Autodesk Fusion 360 part; units mm, degrees
(part 2 of 2)
sketch "Sketch1" plane through (0, 0, 0) normal (0, 0, 1) x (1, 0, 0) in component "Up  Cover - Back"
  line L0 (64, 138) -> (-64, 138)
  line L1 (-64, 138) -> (-64, -138)
  line L2 (-64, -138) -> (64, -138)
  line L3 (64, -138) -> (64, 138)
  line L4 (64, 138) -> (-64, -138) construction
  line L5 (-64, 138) -> (64, -138) construction
  line L6 (-64, 138) -> (-74, 138)
  line L7 (-74, 138) -> (-74, -138)
  line L8 (-74, -138) -> (-64, -138)
  line L9 (-64, -138) -> (-64, 138)
  line L10 (64, 138) -> (87.5, 138)
  line L11 (87.5, 138) -> (87.5, -138)
  line L12 (87.5, -138) -> (64, -138)
  line L13 (64, -138) -> (64, 138)
  circle A0 centre (-74, 0) radius 15
  line L14 (14, 138) -> (64, 88)
  line L15 (64, -88) -> (14, -138)
  line L16 (-74, -138) -> (87.5, -138)
  line L17 (87.5, -138) -> (87.5, -162)
  line L18 (87.5, -162) -> (-74, -162)
  line L19 (-74, -162) -> (-74, -138)
  line L20 (-74, 138) -> (87.5, 138)
  line L21 (87.5, 138) -> (87.5, 162)
  line L22 (87.5, 162) -> (-74, 162)
  line L23 (-74, 162) -> (-74, 138)
  dimension "d3" = 10
  dimension "d4" = 23.5
  dimension "d5" = 30
  dimension "d6" = 50
  dimension "d7" = 50
  dimension "d8" = 50
  dimension "d9" = 50
  dimension "d14" = 161.5
  dimension "d15" = 24
  dimension "d16" = 24
  dimension "d17" = 324
  constraint horizontal L0
  constraint perpendicular L0 L1
  constraint parallel L0 L2
  constraint parallel L1 L3
  constraint coincident L4 origin
  constraint coincident L5 origin
  constraint horizontal L6
  constraint vertical L7
  constraint horizontal L8
  constraint vertical L9
  constraint coincident L1.end L2.start
  constraint horizontal L10
  constraint vertical L11
  constraint horizontal L12
  constraint vertical L13
  constraint coincident L2.end L3.start
  constraint midpoint L7 A0.centre
  constraint coincident L0 L14.start
  constraint coincident L3 L14.end
  constraint coincident L3 L15.start
  constraint coincident L2 L15.end
  constraint horizontal L16
  constraint vertical L17
  constraint horizontal L18
  constraint vertical L19
  constraint coincident L11.end L12.start
  constraint horizontal L20
  constraint vertical L21
  constraint horizontal L22
  constraint vertical L23
  constraint coincident L10.end L11.start
  measures "d3" distance of L0.end L6.end
  measures "d4" distance of L0.start L10.end
  measures "d5" diameter of A0
  measures "d6" distance of L2.end L15.end
  measures "d7" distance of L2.end L15.start
  measures "d8" distance of L0.start L14.end
  measures "d9" distance of L0.start L14.start
  measures "d14" distance of L6.end L10.end
  measures "d15" distance of L11.end L17.end
  measures "d16" distance of L10.end L21.end
  measures "d17" distance of L18.end L22.end
extrude "Extrude1" add sketch "Sketch1" against normal blind 3 contours L0 L3 L13 L14 L20 | L3 L10 L11 L12 L13 L16 L20 | L0 L6 L10 L20 L21 L22 L23 | L0 L1 L2 L3 L9 L13 A0 L14 L15 L16 L20 | L1 L6 L7 L9 A0 L20 | L2 L3 L13 L15 L16 | L2 L8 L12 L16 L17 L18 L19 | L1 L7 L8 L9 A0 L16 makes body 1 in component "Up  Cover - Back"
extrude "Extrude2" add sketch "Sketch1" along normal blind 5 contours L0 L1 L2 L3 L9 L13 A0 L14 L15 L16 L20 bodies 1 in component "Up  Cover - Back"
sketch "Sketch2" plane through (0, 0, 5) normal (0, 0, 1) x (-1, 0, 0) in component "Up  Cover - Back"
  line L0 (-14, -138) -> (64, -138)
  line L1 (64, -138) -> (64, -11.1803)
  arc A0 (64, 11.1803) -> (64, -11.1803) centre (74, 0) ccw
  line L2 (64, 11.1803) -> (64, 138)
  line L3 (64, 138) -> (-14, 138)
  line L4 (-14, 138) -> (-64, 88)
  line L5 (-64, 88) -> (-64, -88)
  line L6 (-64, -88) -> (-14, -138)
  line L7 (59.8579, -5) -> (-64, -5)
  line L8 (59.8579, 5) -> (-64, 5)
  line L9 (-64, -5) -> (-60, -5)
  line L10 (-60, -5) -> (-60, -25)
  line L11 (-60, -25) -> (-64, -25)
  line L12 (-64, -25) -> (-64, -5)
  line L13 (59.8579, -5) -> (55.8579, -5)
  line L14 (55.8579, -5) -> (55.8579, -25)
  line L15 (55.8579, -25) -> (59.8579, -25)
  line L16 (59.8579, -25) -> (59.8579, -5)
  line L17 (55.8579, -15) -> (-60, -15) construction
  line L18 (-4.0711, -5) -> (-0.0711, -5)
  line L19 (-0.0711, -5) -> (-0.0711, -25)
  line L20 (-0.0711, -25) -> (-4.0711, -25)
  line L21 (-4.0711, -25) -> (-4.0711, -5)
  line L22 (-4.0711, -5) -> (-0.0711, -25) construction
  line L23 (-0.0711, -5) -> (-4.0711, -25) construction
  line L24 (59, 0) -> (-64, 0) construction
  line L25 (59.8579, 5) -> (55.8579, 5)
  line L26 (55.8579, 25) -> (59.8579, 25)
  line L27 (59.8579, 25) -> (59.8579, 5)
  line L28 (55.8579, 5) -> (55.8579, 25)
  line L29 (-0.0711, 5) -> (-0.0711, 25)
  line L30 (-0.0711, 25) -> (-4.0711, 25)
  line L31 (-4.0711, 5) -> (-0.0711, 5)
  line L32 (-4.0711, 25) -> (-4.0711, 5)
  line L33 (-64, 5) -> (-60, 5)
  line L34 (-60, 25) -> (-64, 25)
  line L35 (-64, 25) -> (-64, 5)
  line L36 (-60, 5) -> (-60, 25)
  point P0 (-2.0711, -15)
  dimension "d18" = 5
  dimension "d19" = 5
  dimension "d20" = 20
  dimension "d21" = 4
  dimension "d22" = 4
  dimension "d23" = 20
  dimension "d24" = 4
  dimension "d25" = 20
  constraint coincident A0 L7.start
  constraint coincident L5 L7.end
  constraint perpendicular L5 L7
  constraint coincident A0 L8.start
  constraint coincident L5 L8.end
  constraint perpendicular L5 L8
  constraint horizontal L9
  constraint vertical L10
  constraint horizontal L11
  constraint vertical L12
  constraint horizontal L13
  constraint vertical L14
  constraint horizontal L15
  constraint vertical L16
  constraint midpoint L14 L17.start
  constraint midpoint L10 L17.end
  constraint horizontal L18
  constraint perpendicular L18 L19
  constraint parallel L18 L20
  constraint parallel L19 L21
  constraint coincident L22 P0
  constraint coincident L23 P0
  constraint midpoint L17 P0
  constraint midpoint A0 L24.start
  constraint midpoint L5 L24.end
  constraint symmetric L7.start L24 L8.start
  constraint symmetric L7.end L24 L8.end
  constraint symmetric L9.end L24 L33.end
  constraint symmetric L10.end L24 L34.start
  constraint symmetric L11.end L24 L34.end
  constraint symmetric L13.end L24 L25.end
  constraint symmetric L14.end L24 L26.start
  constraint symmetric L15.end L24 L26.end
  constraint symmetric L18.start L24 L31.start
  constraint symmetric L18.end L24 L29.start
  constraint symmetric L19.end L24 L29.end
  constraint symmetric L20.end L24 L30.end
  measures "d18" vertical distance of origin L8.end
  measures "d19" vertical distance of origin L7.end
  measures "d20" distance of L7.end L11.end
  measures "d21" distance of L10.end L11.end
  measures "d22" distance of L7.start L13.end
  measures "d23" distance of L7.start L15.end
  measures "d24" distance of L19.end L20.end
  measures "d25" distance of L18.end L19.end
extrude "Extrude3" add sketch "Sketch2" along normal blind 20 contours L5 L7 L9 L10 L11 L12 | A0 L5 L7 L8 L9 L13 L18 L25 L31 L33 | L7 L13 L14 L15 L16 | L8 L25 L26 L27 L28 | L5 L8 L33 L34 L35 L36 | L7 L18 L19 L20 L21 | L8 L29 L30 L31 L32 bodies 1 in component "Up  Cover - Back"
chamfer "Chamfer1" distance 20 angle 45 6 edges at (-57.8579, -25, 25) (-57.8579, 25, 25) (2.0711, -25, 25) (2.0711, 25, 25) (62, 25, 25) (62, -25, 25) on bodies 1 in component "Up  Cover - Back"
sketch "Sketch3" plane through (0, -5, 0) normal (0, -1, 0) x (1, 0, 0) in component "Up  Cover - Back"
  line L0 (-55.8579, 5) -> (0.0711, 5)
  line L1 (0.0711, 5) -> (0.0711, 25)
  line L2 (0.0711, 25) -> (-55.8579, 25)
  line L3 (-55.8579, 25) -> (-55.8579, 5)
  line L4 (4.0711, 5) -> (60, 5)
  line L5 (60, 5) -> (60, 25)
  line L6 (60, 25) -> (4.0711, 25)
  line L7 (4.0711, 25) -> (4.0711, 5)
  line L8 (-55.8579, 15) -> (60, 15) construction
  circle A0 centre (-49.8579, 15) radius 2.1
  circle A1 centre (-15.8579, 15) radius 2.1
  circle A2 centre (20, 15) radius 2.1
  line L9 (32.0355, 25) -> (32.0355, 5) construction
  line L10 (-27.8934, 25) -> (-27.8934, 5) construction
  circle A3 centre (54, 15) radius 2.1
  line L11 (-59.8579, 25) -> (-59.8579, 5)
  line L12 (64, 5) -> (64, 25)
  dimension "d29" = 4.2
  dimension "d30" = 4.2
  dimension "d31" = 4.2
  dimension "d32" = 4.2
  dimension "d33" = 10
  dimension "d34" = 10
  dimension "d35" = 34
  dimension "d36" = 34
  constraint midpoint L3 L8.start
  constraint midpoint L5 L8.end
  constraint coincident L8 A0.centre
  constraint coincident L8 A1.centre
  constraint coincident L8 A2.centre
  constraint midpoint L6 L9.start
  constraint midpoint L4 L9.end
  constraint midpoint L2 L10.start
  constraint midpoint L0 L10.end
  constraint coincident L8 A3.centre
  measures "d29" diameter of A0
  measures "d30" diameter of A1
  measures "d32" diameter of A3
  measures "d33" distance of A0.centre L11
  measures "d34" distance of A3.centre L12
  measures "d35" distance of A0.centre A1.centre
  measures "d36" distance of A2.centre A3.centre
extrude "Extrude4" cut sketch "Sketch3" against normal through all contours A0 | A1 | A2 | A3 bodies 1 in component "Up  Cover - Back"
split "Split1" by plane through (0, 0, 0) normal (0, 1, 0) bodies 1 makes body 2 at (-16.8924, 111.7787, -3) in component "Up  Cover - Back"
component "Up  Cover - Back" placed x (1, 0, 0) y (0, 1, 0) z (0, 0, 1) at (0, 0, 0)
named bodies: "Up  Cover - Back Right", "Up  Cover - Back Left"

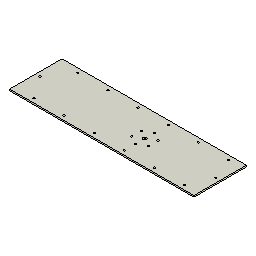
design "Side Cover"
Autodesk Fusion 360 part; units mm, degrees
sketch "Sketch2" plane through (0, 0, 0) normal (0, 0, 1) x (1, 0, 0)
  line L0 (-214.5, -61) -> (-214.5, 61)
  line L1 (-214.5, -61) -> (214.5, 61) construction
  line L2 (-214.5, 61) -> (214.5, 61)
  circle A0 centre (42.5, -3.3) radius 4.1
  line L3 (214.5, -61) -> (-214.5, 61) construction
  line L4 (214.5, 61) -> (214.5, -61)
  line L5 (214.5, -61) -> (-214.5, -61)
  line L6 (-214.5, 0) -> (214.5, 0) construction
  line L7 (-214.5, -3.3) -> (214.5, -3.3) construction
  line L8 (42.5, 61) -> (42.5, -61) construction
  circle A1 centre (42.5, 51) radius 2.1
  line L9 (-214.5, 51) -> (214.5, 51) construction
  circle A2 centre (42.5, -3.3) radius 22.5 construction
  circle A3 centre (42.5, 19.2) radius 2.1
  circle A4 centre (23.0144, 7.95) radius 2.1
  circle A5 centre (23.0144, -14.55) radius 2.1
  circle A6 centre (42.5, -25.8) radius 2.1
  circle A7 centre (61.9856, -14.55) radius 2.1
  circle A8 centre (61.9856, 7.95) radius 2.1
  line L10 (-194.5, 61) -> (-194.5, -61) construction
  line L11 (194.5, 61) -> (194.5, -61) construction
  circle A9 centre (-167.5, 51) radius 2.1
  circle A10 centre (-97.5, 51) radius 2.1
  circle A11 centre (-27.5, 51) radius 2.1
  circle A12 centre (112.5, 51) radius 2.1
  circle A13 centre (182.5, 51) radius 2.1
  circle A14 centre (112.5, -51) radius 2.1
  line L12 (-214.5, -51) -> (214.5, -51) construction
  circle A15 centre (-27.5, -51) radius 2.1
  circle A16 centre (-167.5, -51) radius 2.1
  circle A17 centre (182.5, -51) radius 2.1
  circle A18 centre (-97.5, -51) radius 2.1
  circle A19 centre (42.5, -51) radius 2.1
  circle A20 centre (-204.5, 0) radius 2.1
  circle A21 centre (204.5, 0) radius 2.1
  dimension "d11" = 122
  dimension "d12" = 429
  dimension "d14" = 8.2
  dimension "d18" = 3.3
  dimension "d20" = 172
  dimension "d21" = 4.2
  dimension "d23" = 10
  dimension "d24" = 45
  dimension "d25" = 4.2
  dimension "d27" = 360
  dimension "d30" = 70
  dimension "d31" = 0
  dimension "d32" = 20
  dimension "d33" = 20
  dimension "d34" = 4.2
  dimension "d35" = 10
  dimension "d36" = 4.2
  dimension "d37" = 10
  constraint perpendicular L0 L5
  constraint parallel L2 L5
  constraint parallel L0 L4
  constraint horizontal L5
  constraint coincident origin L3
  constraint coincident origin L1
  constraint midpoint L0 L6.start
  constraint midpoint L4 L6.end
  constraint coincident A0.centre L7
  constraint coincident L2 L8.start
  constraint coincident L5 L8.end
  constraint perpendicular L5 L8
  constraint coincident A0.centre L8
  constraint coincident L8 A1.centre
  constraint coincident L0 L9.start
  constraint coincident L4 L9.end
  constraint perpendicular L4 L9
  constraint coincident A1.centre L9
  constraint concentric A0 A2
  constraint coincident A2 A3.centre
  constraint coincident L8 A3.centre
  constraint coincident L2 L10.start
  constraint coincident L5 L10.end
  constraint perpendicular L5 L10
  constraint coincident L2 L11.start
  constraint coincident L5 L11.end
  constraint perpendicular L5 L11
  constraint symmetric L6 A1 A19
  constraint symmetric L6 L9.start L12.start
  constraint symmetric L6 L9.end L12.end
  constraint symmetric L6 A9 A16
  constraint symmetric L6 A10 A18
  constraint symmetric L6 A11 A15
  constraint symmetric L6 A12 A14
  constraint symmetric L6 A13 A17
  constraint coincident L6 A20.centre
  constraint coincident L6 A21.centre
  measures "d11" distance of L0.start L0.end
  measures "d12" distance of L0.end L1.end
  measures "d14" diameter of A0
  measures "d20" distance of L1.end L8.start
  measures "d21" diameter of A1
  measures "d23" distance of L1.end L9.end
  measures "d24" diameter of A2
  measures "d25" diameter of A3
  measures "d32" distance of L0 L10
  measures "d33" distance of L4 L11
  measures "d34" diameter of A20
  measures "d35" distance of L6.start A20.centre
  measures "d36" diameter of A21
  measures "d37" distance of L6.end A21.centre
extrude "Extrude2" add sketch "Sketch2" along normal blind 3.5
sketch "Sketch3" plane through (0, 0, 3.5) normal (0, 0, 1) x (-1, 0, 0)
  circle A0 centre (-42.5, 3.3) radius 4
  line L0 (-214.5, 61) -> (-214.5, -61)
  line L1 (-214.5, -61) -> (214.5, -61)
  line L2 (214.5, -61) -> (214.5, 61)
  line L3 (214.5, 61) -> (-214.5, 61)
  line L4 (-130, -50) -> (-141.5967, -50) construction
  line L5 (-141.5967, -50) -> (-141.5967, -60) construction
  line L6 (-141.5967, -60) -> (-130, -60) construction
  line L7 (-130, -60) -> (-130, -50) construction
  circle A1 centre (-182.5, 51) radius 2.1
  circle A2 centre (97.5, 51) radius 2.1
  circle A3 centre (-42.5, 51) radius 2.1
  circle A4 centre (204.5, 0) radius 2.1
  circle A5 centre (-204.5, 0) radius 2.1
  circle A6 centre (167.5, 51) radius 2.1
  circle A7 centre (97.5, -51) radius 2.1
  circle A8 centre (27.5, -51) radius 2.1
  circle A9 centre (-112.5, -51) radius 2.1
  circle A10 centre (-182.5, -51) radius 2.1
  circle A11 centre (-112.5, 51) radius 2.1
  circle A12 centre (27.5, 51) radius 2.1
  circle A13 centre (167.5, -51) radius 2.1
  circle A14 centre (-61.9856, -7.95) radius 2.1
  circle A15 centre (-61.9856, 14.55) radius 2.1
  circle A16 centre (-42.5, 25.8) radius 2.1
  circle A17 centre (-23.0144, 14.55) radius 2.1
  circle A18 centre (-23.0144, -7.95) radius 2.1
  circle A19 centre (-42.5, -19.2) radius 2.1
  circle A20 centre (-42.5, -51) radius 2.1
  circle A21 centre (-42.5, 3.3) radius 4.1
  line L8 (-214.5, 61) -> (-214.5, -61)
  line L9 (-214.5, -61) -> (214.5, -61)
  line L10 (214.5, -61) -> (214.5, 61)
  line L11 (214.5, 61) -> (-214.5, 61)
  constraint perpendicular L4 L5
  constraint parallel L4 L6
  constraint parallel L5 L7

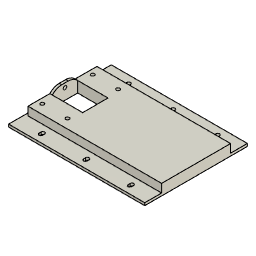
design "Back Cover"
Autodesk Fusion 360 part; units mm, degrees
sketch "Sketch1" plane through (0, 0, 0) normal (0, 0, 1) x (1, 0, 0)
  line L0 (-79.25, 60.9) -> (79.25, 60.9)
  line L1 (79.25, 60.9) -> (79.25, -60.9)
  line L2 (79.25, -60.9) -> (-79.25, -60.9)
  line L3 (-79.25, -60.9) -> (-79.25, 60.9)
  line L4 (-79.25, 60.9) -> (79.25, -60.9) construction
  line L5 (79.25, 60.9) -> (-79.25, -60.9) construction
  line L6 (79.25, -40.9) -> (-79.25, -40.9)
  line L7 (-79.25, -40.9) -> (-79.25, 40.9)
  line L8 (-79.25, 40.9) -> (79.25, 40.9)
  line L9 (79.25, 40.9) -> (79.25, -40.9)
  line L10 (79.25, -40.9) -> (-79.25, 40.9) construction
  line L11 (-79.25, -40.9) -> (79.25, 40.9) construction
  line L12 (0, 0) -> (0, 60.9) construction
  line L13 (-79.25, 60.9) -> (79.25, 40.9) construction
  line L14 (0, 50.9) -> (-79.25, 50.9) construction
  line L15 (0, 50.9) -> (79.25, 50.9) construction
  line L16 (-2.1, 52.15) -> (-2.1, 49.65)
  arc A0 (-2.1, 49.65) -> (2.1, 49.65) centre (0, 49.65) ccw
  line L17 (2.1, 49.65) -> (2.1, 52.15)
  arc A1 (2.1, 52.15) -> (-2.1, 52.15) centre (0, 52.15) ccw
  line L18 (0, 52.15) -> (0, 49.65) construction
  arc A2 (-50.7333, 52.15) -> (-54.9333, 52.15) centre (-52.8333, 52.15) ccw
  line L19 (-54.9333, 52.15) -> (-54.9333, 49.65)
  arc A3 (-54.9333, 49.65) -> (-50.7333, 49.65) centre (-52.8333, 49.65) ccw
  line L20 (-50.7333, 49.65) -> (-50.7333, 52.15)
  arc A4 (54.9333, 52.15) -> (50.7333, 52.15) centre (52.8333, 52.15) ccw
  line L21 (50.7333, 52.15) -> (50.7333, 49.65)
  arc A5 (50.7333, 49.65) -> (54.9333, 49.65) centre (52.8333, 49.65) ccw
  line L22 (54.9333, 49.65) -> (54.9333, 52.15)
  line L23 (-79.25, 0) -> (79.25, 0) construction
  arc A6 (-54.9333, -52.15) -> (-50.7333, -52.15) centre (-52.8333, -52.15) ccw
  line L24 (-54.9333, -52.15) -> (-54.9333, -49.65)
  arc A7 (-50.7333, -49.65) -> (-54.9333, -49.65) centre (-52.8333, -49.65) ccw
  line L25 (-50.7333, -49.65) -> (-50.7333, -52.15)
  arc A8 (-2.1, -52.15) -> (2.1, -52.15) centre (0, -52.15) ccw
  line L26 (-2.1, -52.15) -> (-2.1, -49.65)
  line L27 (2.1, -49.65) -> (2.1, -52.15)
  arc A9 (2.1, -49.65) -> (-2.1, -49.65) centre (0, -49.65) ccw
  arc A10 (50.7333, -52.15) -> (54.9333, -52.15) centre (52.8333, -52.15) ccw
  line L28 (50.7333, -52.15) -> (50.7333, -49.65)
  line L29 (54.9333, -49.65) -> (54.9333, -52.15)
  arc A11 (54.9333, -49.65) -> (50.7333, -49.65) centre (52.8333, -49.65) ccw
  line L30 (-2.1, 50.9) -> (2.1, 50.9) construction
  line L31 (-37.25, 40.9) -> (-37.25, -40.9) construction
  line L32 (-40.25, 15) -> (-76.25, 15)
  line L33 (-76.25, 15) -> (-76.25, -15)
  line L34 (-76.25, -15) -> (-40.25, -15)
  line L35 (-40.25, -15) -> (-40.25, 15)
  line L36 (-40.25, 15) -> (-76.25, -15) construction
  line L37 (-76.25, 15) -> (-40.25, -15) construction
  line L38 (-43.25, -30) -> (-73.25, -30) construction
  line L39 (-73.25, -30) -> (-73.25, 30) construction
  line L40 (-73.25, 30) -> (-43.25, 30) construction
  line L41 (-43.25, 30) -> (-43.25, -30) construction
  line L42 (-43.25, -30) -> (-73.25, 30) construction
  line L43 (-73.25, -30) -> (-43.25, 30) construction
  circle A12 centre (-73.25, -30) radius 2.1
  circle A13 centre (-43.25, -30) radius 2.1
  circle A14 centre (-73.25, 30) radius 2.1
  circle A15 centre (-43.25, 30) radius 2.1
  line L44 (-79.25, 60.9) -> (-82.25, 60.9)
  line L45 (-82.25, 60.9) -> (-82.25, -60.9)
  line L46 (-82.25, -60.9) -> (-79.25, -60.9)
  line L47 (-79.25, -60.9) -> (-79.25, 60.9)
  point P0 (-58.25, 0)
  point P1 (-58.25, 0)
  dimension "d1" = 121.8
  dimension "d2" = 158.5
  dimension "d3" = 81.8
  dimension "d13" = 4.2
  dimension "d14" = 2.5
  dimension "d22" = 52.8333
  dimension "d23" = 0
  dimension "d26" = 42
  dimension "d27" = 36
  dimension "d28" = 30
  dimension "d29" = 3
  dimension "d30" = 30
  dimension "d31" = 60
  dimension "d32" = 4.2
  dimension "d33" = 4.2
  dimension "d34" = 4.2
  dimension "d35" = 4.2
  dimension "d40" = 3
  constraint perpendicular L0 L1
  constraint parallel L0 L2
  constraint perpendicular L6 L7
  constraint parallel L6 L8
  constraint horizontal L6
  constraint coincident L1 L6.start
  constraint midpoint L0 L12.end
  constraint midpoint L13 L14.start
  constraint coincident L3 L14.end
  constraint perpendicular L3 L14
  constraint coincident L1 L15.end
  constraint perpendicular L1 L15
  constraint tangent L16 A0
  constraint tangent A0 L17
  constraint parallel L16 L17
  constraint tangent L17 A1
  constraint tangent L16 A1
  constraint perpendicular L14 L18
  constraint coincident L12.start L4
  constraint midpoint L12.start L4
  constraint midpoint L12.start L5
  constraint midpoint L12.start L10
  constraint midpoint L12.start L11
  constraint coincident L12.start origin
  constraint coincident L12 A1.centre
  constraint midpoint L3 L23.start
  constraint midpoint L1 L23.end
  constraint symmetric L16.start L23 A8.start
  constraint symmetric L16.end L23 L26.end
  constraint symmetric A0.end L23 L27.start
  constraint symmetric L17.end L23 A8.end
  constraint symmetric A0 L23 A9
  constraint symmetric A1 L23 A8
  constraint symmetric A2.start L23 A6.end
  constraint symmetric A2.end L23 A6.start
  constraint symmetric A2 L23 A6
  constraint symmetric L19.end L23 L24.end
  constraint symmetric A3.end L23 A7.start
  constraint symmetric A3 L23 A7
  constraint symmetric A4.start L23 A10.end
  constraint symmetric A4.end L23 A10.start
  constraint symmetric A4 L23 A10
  constraint symmetric L21.end L23 L28.end
  constraint symmetric A5.end L23 L29.start
  constraint symmetric A5 L23 A11
  constraint midpoint L16 L30.start
  constraint midpoint L17 L30.end
  constraint coincident L14.start L30
  constraint coincident L8 L31.start
  constraint coincident L6 L31.end
  constraint perpendicular L6 L31
  constraint horizontal L32
  constraint perpendicular L32 L33
  constraint parallel L32 L34
  constraint parallel L33 L35
  constraint coincident L36 P1
  constraint coincident L37 P1
  constraint coincident L23 P1
  constraint horizontal L38
  constraint perpendicular L38 L39
  constraint parallel L38 L40
  constraint parallel L39 L41
  constraint coincident L42 P1
  constraint coincident L43 P1
  constraint coincident P1 P0
  constraint coincident L38.end L39.start
  constraint coincident L38.start L41.end
  constraint coincident L39.end L40.start
  constraint coincident L40.end L41.start
  constraint horizontal L44
  constraint vertical L45
  constraint horizontal L46
  constraint vertical L47
  constraint coincident L2.end L3.start
  measures "d1" distance of L0.start L2.end
  measures "d2" distance of L0.start L0.end
  measures "d3" distance of L6.end L7.end
  measures "d13" diameter of A0
  measures "d14" distance of A1.centre A0.centre
  measures "d26" distance of L3 L31
  measures "d27" distance of L33.end L34.end
  measures "d28" distance of L32.end L33.end
  measures "d29" distance of L3 L33
  measures "d30" distance of L39.end L40.end
  measures "d31" distance of L38.end L39.end
  measures "d32" diameter of A12
  measures "d33" diameter of A13
  measures "d34" diameter of A14
  measures "d35" diameter of A15
  measures "d40" distance of L45.end L2.end
extrude "Extrude1" add sketch "Sketch1" along normal blind 9.9 contours L1 L3 L6 L7 L8 L9 L47
extrude "Extrude2" add sketch "Sketch1" against normal blind 3
sketch "Sketch7" plane through (0, 0, 9.9) normal (0, 0, 1) x (-1, 0, 0)
  circle A0 centre (73.25, -30) radius 2.1
  circle A1 centre (43.25, -30) radius 2.1
  circle A2 centre (43.25, 30) radius 2.1
  line L0 (40.25, -15) -> (40.25, 15)
  line L1 (40.25, 15) -> (76.25, 15)
  line L2 (76.25, 15) -> (76.25, -15)
  line L3 (76.25, -15) -> (40.25, -15)
  circle A3 centre (73.25, 30) radius 2.1
  line L4 (-79.25, -40.9) -> (79.25, -40.9)
  line L5 (79.25, -40.9) -> (79.25, 40.9)
  line L6 (79.25, 40.9) -> (-79.25, 40.9)
  line L7 (-79.25, 40.9) -> (-79.25, -40.9)
  line L8 (76.25, -15) -> (79.25, -15)
  line L9 (79.25, -15) -> (79.25, 15)
  line L10 (79.25, 15) -> (76.25, 15)
  line L11 (76.25, 15) -> (76.25, -15)
  constraint horizontal L8
  constraint vertical L9
  constraint horizontal L10
  constraint vertical L11
  constraint coincident L5 L9.end
  constraint coincident L2.end L3.start
extrude "Extrude5" add sketch "Sketch7" along normal blind 5 contours L2 L5 L8 L9 L10 L11
fillet "Fillet1" radius 15 2 edges at (-77.75, 15, 14.9) (-77.75, -15, 14.9)
sketch "Sketch6" plane through (-79.25, 0, 0) normal (-1, 0, 0) x (0, -1, 0)
  line L0 (40.9, 0) -> (40.9, 9.9)
  line L1 (-15, 9.9) -> (-40.9, 9.9)
  line L2 (-40.9, 9.9) -> (-40.9, 0)
  line L3 (-40.9, 0) -> (40.9, 0)
  line L4 (0, 0) -> (0, 10) construction
  circle A0 centre (0, 10) radius 2.1
  arc A1 (15, 9.9) -> (3.8197, 14.9) centre (3.8197, -0.1) ccw
  line L5 (3.8197, 14.9) -> (-3.8197, 14.9)
  arc A2 (-3.8197, 14.9) -> (-15, 9.9) centre (-3.8197, -0.1) ccw
  line L6 (40.9, 9.9) -> (15, 9.9)
  dimension "d36" = 10
  dimension "d37" = 4.2
  constraint coincident L4.start origin
  constraint vertical L4
  constraint coincident L4.end A0.centre
  measures "d36" distance of L4.start L4.end
  measures "d37" diameter of A0
extrude "Extrude4" cut sketch "Sketch6" against normal blind 6 contours A0
equation "d2 = ( 317 / 2 ) * 1 mm"
equation "d22 = ( 158.5 / 3 ) * 1 mm"
equation "d26 = 45 mm - 3 mm"
